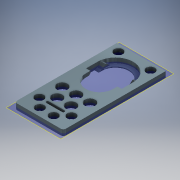
# Autodesk Inventor part: Cup_Dispenser_Slider
Saved by Autodesk Inventor 2016 (Build 200138000, 138)
## iProperties
Created: 2015-07-09
Part Number: Cup_Dispenser_Slider
Material: Generic
Document SubType Name: Modeling
Designer: marku
Density: 1 g/cm^3
Appearance: Lead
Author: marku
Autodesk Inventor part; units mm, degrees
ref_plane "YZ Plane" through (0, 0, 0) normal (1, 0, 0) x (0, 1, 0)
ref_plane "XZ Plane" through (0, 0, 0) normal (0, 1, 0) x (-1, 0, 0)
ref_plane "XY Plane" through (0, 0, 0) normal (0, 0, 1) x (1, 0, 0)
sketch "Sketch2" plane through (0, 0, 0) normal (0, 0, 1) x (1, 0, 0)
  line L0 (57, 57.2078) -> (57, 117.2078) projected
  line L1 (57, -62.7922) -> (57, 57.2078) projected
  line L2 (57, -112.7922) -> (57, -62.7922) projected
  arc A0 (50, -119.7922) -> (57, -112.7922) centre (50, -112.7922) ccw projected
  line L3 (0, -119.7922) -> (50, -119.7922) projected
  line L4 (-50, -119.7922) -> (0, -119.7922) projected
  arc A1 (-57, -112.7922) -> (-50, -119.7922) centre (-50, -112.7922) ccw projected
  line L5 (-57, -62.7922) -> (-57, -112.7922) projected
  line L6 (-57, 57.2078) -> (-57, -62.7922) projected
  line L7 (-57, 117.2078) -> (-57, 57.2078) projected
  line L8 (-57, 117.2078) -> (57, 117.2078) projected
  line L9 (54, 114.2078) -> (54, 57.2078)
  line L10 (54, 57.2078) -> (54, -62.7922)
  line L11 (54, -62.7922) -> (54, -112.7922)
  arc A2 (50, -116.7922) -> (54, -112.7922) centre (50, -112.7922) ccw
  line L12 (50, -116.7922) -> (0, -116.7922)
  line L13 (0, -116.7922) -> (-50, -116.7922)
  arc A3 (-54, -112.7922) -> (-50, -116.7922) centre (-50, -112.7922) ccw
  line L14 (-54, -112.7922) -> (-54, -62.7922)
  line L15 (-54, -62.7922) -> (-54, 57.2078)
  line L16 (-54, 57.2078) -> (-54, 114.2078)
  line L17 (-54, 114.2078) -> (54, 114.2078)
  point P0 (0, 0)
  dimension "d5" = 3
  constraints: 18 end point, 4 point on circle, 2 centre point, 10 other
  measures "d5" distance between parallel lines of L0 L9
ref_plane "Work Plane1" through (-57, -119.7922, 15) normal (0, 0, -1) x (0, 1, 0)
extrude "Extrusion1" add sketch "Sketch2" along normal up to surface (15 mm away)
sketch "Sketch3" plane through (0, 0, 0) normal (0, 0, -1) x (-1, 0, 0)
  circle A0 centre (0, 57.2078) radius 57 construction
  arc A1 (31.25, 57.2078) -> (-31.25, 57.2078) centre (0, 57.2078) ccw
  line L0 (-54, -112.7922) -> (-54, 114.2078) projected
  line L1 (-54, 114.2078) -> (54, 114.2078) projected
  line L2 (54, 114.2078) -> (54, -112.7922) projected
  line L3 (-31.25, 57.2078) -> (-31.25, 47.2078)
  line L4 (-31.25, 47.2078) -> (-54, 47.2078)
  line L5 (31.25, 57.2078) -> (31.25, 47.2078)
  line L6 (31.25, 47.2078) -> (54, 47.2078)
  point P0 (0, 0)
  dimension "d8" = 31.25
  dimension "d9" = 10
  dimension "d10" = 10
  constraints: 8 end point, 4 point on line, 2 perpendicular, 2 point on circle, 1 centre point, 1 coincident, 1 tangent, 1 vertical
  measures "d8" radius of A1
  measures "d9" distance of L3.start L3.end
  measures "d10" distance of L5.start L5.end
extrude "Extrusion2" add sketch "Sketch3" against normal blind 3
ref_plane "Work Plane2" through (0, 0, 6) normal (0, 0, -1) x (-1, 0, 0)
sketch "Sketch4" plane through (0, 0, 6) normal (0, 0, -1) x (-1, 0, 0)
  line L0 (-54, -112.7922) -> (-54, 47.2078) projected
  arc A0 (-54, -112.7922) -> (-50, -116.7922) centre (-50, -112.7922) ccw projected
  line L1 (50, -116.7922) -> (-50, -116.7922) projected
  arc A1 (50, -116.7922) -> (54, -112.7922) centre (50, -112.7922) ccw projected
  line L2 (54, 47.2078) -> (54, -112.7922) projected
  line L3 (0, -163.3413) -> (0, 169.6733) construction
  line L4 (-31.25, 47.2078) -> (-54, 47.2078) construction
  circle A2 centre (0, 20.6666) radius 41 construction
  arc A3 (-31.25, 20.6666) -> (31.25, 20.6666) centre (0, 20.6666) ccw
  line L5 (-31.25, 20.6666) -> (-31.25, 30.6666)
  line L6 (31.25, 20.6666) -> (31.25, 30.6666)
  line L7 (31.25, 30.6666) -> (54, 30.6666)
  line L8 (-31.25, 30.6666) -> (-54, 30.6666)
  point P0 (0, 0)
  dimension "d14" = 82
  dimension "d15" = 10
  dimension "d16" = 31.25
  constraints: 10 end point, 4 point on line, 3 vertical, 2 perpendicular, 2 point on circle, 2 tangent, 1 centre point, 1 coincident, 1 parallel, 3 other
  measures "d15" distance of L5.start L5.end
  measures "d16" radius of A3
extrude "Extrusion3" add sketch "Sketch4" against normal up to surface (9 mm away)
sketch "Sketch5" plane through (0, 0, 3) normal (0, 0, 1) x (1, 0, 0)
  arc A0 (31.25, 57.2078) -> (-31.25, 57.2078) centre (0, 57.2078) ccw projected
  line L0 (31.25, 57.2078) -> (31.25, 47.2078) projected
  line L1 (31.25, 47.2078) -> (54, 47.2078) projected
  line L2 (54, 114.2078) -> (54, 47.2078) projected
  line L3 (-54, 114.2078) -> (54, 114.2078) projected
  line L4 (-54, 47.2078) -> (-54, 114.2078) projected
  line L5 (-54, 47.2078) -> (-31.25, 47.2078) projected
  line L6 (-31.25, 47.2078) -> (-31.25, 57.2078) projected
  arc A1 (41, 57.2078) -> (-41, 57.2078) centre (0, 57.2078) ccw
  line L7 (41, 57.2078) -> (41, 56.9578)
  line L8 (41, 56.9578) -> (44.25, 56.9578)
  line L9 (44.25, 56.9578) -> (44.25, 104.4578)
  line L10 (44.25, 104.4578) -> (-44.25, 104.4578)
  line L11 (-44.25, 104.4578) -> (-44.25, 56.9578)
  line L12 (-44.25, 56.9578) -> (-41, 56.9578)
  line L13 (-41, 56.9578) -> (-41, 57.2078)
  line L14 (-44.25, 56.9578) -> (-54, 56.9578)
  line L15 (44.25, 56.9578) -> (54, 56.9578)
  point P0 (0, 0)
  dimension "d19" = 41
  constraints: 18 end point, 3 point on line, 2 point on circle, 1 centre point, 1 perpendicular, 7 other
  measures "d19" horizontal distance of A0.centre L12.end
extrude "Extrusion4" add sketch "Sketch5" along normal up to surface (12 mm away) contours L15 L9 L10 L11 L14 L4 L3 L2 | L8 L7 A1 L13 L12 L11 L10 L9
sketch "Sketch6" plane through (0, 0, 6) normal (0, 0, -1) x (-1, 0, 0)
  line L0 (-54, -112.7922) -> (-54, 30.6666) projected
  arc A0 (-54, -112.7922) -> (-50, -116.7922) centre (-50, -112.7922) ccw projected
  line L1 (50, -116.7922) -> (-50, -116.7922) projected
  arc A1 (50, -116.7922) -> (54, -112.7922) centre (50, -112.7922) ccw projected
  line L2 (54, 30.6666) -> (54, -112.7922) projected
  line L3 (31.25, 30.6666) -> (54, 30.6666) projected
  line L4 (31.25, 20.6666) -> (31.25, 30.6666) projected
  arc A2 (-31.25, 20.6666) -> (31.25, 20.6666) centre (0, 20.6666) ccw projected
  line L5 (-31.25, 30.6666) -> (-31.25, 20.6666) projected
  line L6 (-54, 30.6666) -> (-31.25, 30.6666) projected
  line L7 (41, 20.6666) -> (41, 20.9166)
  line L8 (41, 20.9166) -> (44.25, 20.9166)
  line L9 (44.25, 20.9166) -> (44.25, -107.0422)
  line L10 (44.25, -107.0422) -> (-44.25, -107.0422)
  line L11 (-44.25, -107.0422) -> (-44.25, 20.9166)
  line L12 (-44.25, 20.9166) -> (-41, 20.9166)
  line L13 (-41, 20.9166) -> (-41, 20.6666)
  arc A3 (-41, 20.6666) -> (41, 20.6666) centre (0, 20.6666) ccw
  line L14 (44.25, 20.9166) -> (54, 20.9166)
  line L15 (-44.25, 20.9166) -> (-54, 20.9166)
  point P0 (0, 0)
  dimension "d22" = 41
  constraints: 18 end point, 3 point on line, 2 point on circle, 1 centre point, 1 perpendicular, 7 other
  measures "d22" distance of A2.centre L7.start
extrude "Extrusion5" add sketch "Sketch6" along normal up to surface (6 mm away) contours L0 L15 L11 L10 L9 L14 L2 A1 L1 A0 | L12 L13 A3 L7 L8 L9 L10 L11
sketch "Sketch7" plane through (0, 0, 0) normal (0, 0, -1) x (-1, 0, 0)
  line L0 (54, 20.9166) -> (41, 20.9166) projected
  line L1 (41, 20.9166) -> (54, 20.9166) projected
  line L2 (54, 56.9578) -> (41, 56.9578) projected
  line L3 (41, 56.9578) -> (54, 56.9578) projected
  line L4 (54, 47.2078) -> (54, 20.9166) projected
  line L5 (54, 56.9578) -> (54, 20.9166)
  line L6 (41, 56.9578) -> (41, 20.9166)
  line L7 (-41, 56.9578) -> (-54, 56.9578) projected
  line L8 (-41, 20.9166) -> (-54, 20.9166) projected
  line L9 (-41, 56.9578) -> (-41, 20.9166)
  line L10 (-54, 20.9166) -> (-54, 47.2078) projected
  line L11 (-54, 56.9578) -> (-54, 20.9166)
  point P0 (0, 0)
  constraints: 8 end point, 2 collinear, 2 vertical
extrude "Extrusion6" add sketch "Sketch7" against normal up to surface (15 mm away)
chamfer "Chamfer1" distance 10 distance2 3 1 edges at (36.125, 47.2078, 3) measured on face at (36.125, 47.7078, 3)
chamfer "Chamfer2" distance 10 distance2 3 1 edges at (-36.125, 47.2078, 3) measured on face at (-36.125, 47.7078, 3)
sketch "Sketch9" plane through (41, 30.6666, 15) normal (-1, 0, 0) x (0, 0, 1)
  line L0 (-15, 16.5412) -> (-12, 26.5412) projected
  line L1 (-12, 26.5412) -> (-12, 67.5412) projected
  line L2 (-12, 26.5412) -> (-4, 36.0753)
  line L3 (-4, 36.0753) -> (-12, 45.6093)
  line L4 (-12, 26.5412) -> (-12, 45.6093)
  line L5 (-4, 36.0753) -> (-12, 36.0753) construction
  point P0 (-15, -30.6666)
  dimension "d41" = 100
  dimension "d42" = 8
  constraints: 8 end point, 1 collinear, 1 midpoint, 1 point on line, 1 other
  measures "d41" angle of L2 L3
  measures "d42" distance from line of L1 L2.end
extrude "Extrusion8" add sketch "Sketch9" along normal up to surface (9.75 mm away)
mirror "Mirror1" about plane through (0, 0, 0) normal (1, 0, 0) of "Extrusion8"
fillet "Fillet1" radius 2 2 edges at (-35.563, 66.7418, 11) (35.563, 66.7418, 11)
chamfer "Chamfer4" distance 3 angle 45 2 edges at (36.125, 30.6666, 6) (-36.125, 30.6666, 6)
sketch "Sketch8" plane through (-57, 117.2078, 15) normal (0, 0, 1) x (1, 0, 0)
  arc A0 (98, -60) -> (16, -60) centre (57, -60) ccw construction
  arc A1 (16, -96.5412) -> (98, -96.5412) centre (57, -96.5412) ccw construction
  line L0 (57, -60) -> (57, -96.5412) construction
  circle A2 centre (57, -180) radius 57 construction
  line L1 (57, -180) -> (142.4239, -180) construction
  line L2 (57, -161.7294) -> (57, -198.2706) construction
  circle A3 centre (57, -180) radius 18.2706 construction
  line L3 (38.7294, -198.2706) -> (75.2706, -198.2706) construction
  line L4 (38.7294, -201.2706) -> (75.2706, -201.2706)
  line L5 (75.2706, -195.2706) -> (38.7294, -195.2706)
  arc A4 (38.7294, -195.2706) -> (38.7294, -201.2706) centre (38.7294, -198.2706) ccw
  arc A5 (75.2706, -201.2706) -> (75.2706, -195.2706) centre (75.2706, -198.2706) ccw
  line L6 (75.2706, -180) -> (75.2706, -198.2706) construction
  point P0 (57, -117.2078)
  dimension "d33" = 6
  constraints: 16 end point, 6 point on circle, 6 tangent, 3 centre point, 2 horizontal, 2 midpoint, 2 vertical, 1 coincident, 1 collinear, 1 parallel, 1 perpendicular, 1 point on line, 1 symmetric about line
  measures "d33" diameter of A5
extrude "Extrusion7" cut sketch "Sketch8" against normal up to surface (15 mm away)
chamfer "Chamfer3" distance 1.5 angle 45 4 edges at (0, -78.0628, 0) (-21.2706, -81.0628, 0) (0, -84.0628, 0) (21.2706, -81.0628, 0)
sketch "Sketch10" plane through (-57, 117.2078, 0) normal (0, 1, 0) x (1, 0, 0)
  line L0 (0, 0) -> (0, -15) projected
  line L1 (0, -7.5) -> (114, -7.5) construction
  line L2 (114, 0) -> (114, -15) projected
  line L3 (57, 0) -> (57, -7.5) construction
  line L4 (57, -7.5) -> (57, -15) construction
  point P0 (15, -7.5)
  point P1 (99, -7.5)
  dimension "d46" = 15
  constraints: 6 end point, 3 midpoint, 2 point on line, 1 symmetric about line
  measures "d46" distance from line of L0 point (15, -7.5)
hole "Hole1" at (-42, 117.2078, 7.5) at (42, 117.2078, 7.5) direction (0, -1, 0) diameter 3 depth 8 tip angle 118
thicken "Thicken1" operation add thickness 0.8 both sides no extend neighbours yes toward (0, 0, -1) faces at (-51.6667, 11.694, 15) (-57, 40.5411, 5) (57, -36.1255, 5) (-50.5231, -119.7726, 10) (-16.6667, -119.7922, 5) (50.5231, -119.7726, 5) (51.6667, 8.3607, 0)
sketch "Sketch11" plane through (-56.2, 117.2078, 14.2) normal (0, 0, 1) x (1, 0, 0)
  circle A0 centre (56.2, -150.5412) radius 12
  line L0 (74.4706, -201.2706) -> (37.9294, -201.2706) construction
  arc A1 (37.9294, -195.2706) -> (37.9294, -201.2706) centre (37.9294, -198.2706) ccw construction
  line L1 (37.9294, -195.2706) -> (74.4706, -195.2706) construction
  arc A2 (74.4706, -201.2706) -> (74.4706, -195.2706) centre (74.4706, -198.2706) ccw construction
  line L2 (112.4, -230) -> (112.4, 0) construction
  line L3 (112.4, 0) -> (0, 0) construction
  line L4 (0, 0) -> (0, -230) construction
  arc A3 (0, -230) -> (6.2, -236.2) centre (6.2, -230) ccw construction
  line L5 (6.2, -236.2) -> (106.2, -236.2) construction
  arc A4 (106.2, -236.2) -> (112.4, -230) centre (106.2, -230) ccw construction
  line L6 (15.2, -86.5412) -> (15.2, -60) construction
  arc A5 (97.2, -60) -> (15.2, -60) centre (56.2, -60) ccw construction
  line L7 (97.2, -60) -> (97.2, -86.5412) construction
  line L8 (97.2, -86.5412) -> (87.45, -86.5412) construction
  line L9 (87.45, -86.5412) -> (87.45, -96.5412) construction
  arc A6 (24.95, -96.5412) -> (87.45, -96.5412) centre (56.2, -96.5412) ccw construction
  line L10 (24.95, -96.5412) -> (24.95, -86.5412) construction
  line L11 (24.95, -86.5412) -> (15.2, -86.5412) construction
  circle A7 centre (88.2, -150.5412) radius 12
  circle A8 centre (24.2, -150.5412) radius 12
  circle A9 centre (72.2, -178.2541) radius 12
  line L12 (56.2, -150.5412) -> (72.2, -178.2541) construction
  line L13 (72.2, -178.2541) -> (88.2, -150.5412) construction
  line L14 (88.2, -150.5412) -> (56.2, -150.5412) construction
  circle A10 centre (40.2, -178.2541) radius 12
  circle A11 centre (93.2, -198.2706) radius 10
  circle A12 centre (19.2, -198.2706) radius 10
  line L15 (56.2, -60) -> (56.2, -293.0623) construction
  circle A13 centre (72.2, -218.2706) radius 10
  line L16 (72.2, -178.2541) -> (72.2, -218.2706) construction
  circle A14 centre (40.2, -218.2706) radius 10
  circle A15 centre (19.2, -16) radius 10
  circle A16 centre (93.2, -16) radius 10
  line L17 (93.2, -16) -> (93.2, -198.2706) construction
  arc A17 (74.4706, -201.2706) -> (74.4706, -195.2706) centre (74.4706, -198.2706) ccw construction
  line L18 (93.2, -198.2706) -> (74.4706, -198.2706) construction
  point P0 (56.2, -117.2078)
  dimension "d56" = 24
  dimension "d59" = 32
  dimension "d66" = 32
  dimension "d71" = 24
  dimension "d74" = 32
  dimension "d79" = 20
  dimension "d80" = 20
  dimension "d81" = 20
  dimension "d82" = 20
  dimension "d83" = 5
  dimension "d84" = 16
  dimension "d85" = 54
  dimension "d86" = 20
  constraints: 14 end point, 11 centre point, 5 horizontal, 3 symmetric about line, 3 vertical, 2 equal length, 1 point on line, 8 other
  measures "d56" diameter of A0
  measures "d59" distance of L12.start L13.end
  measures "d66" distance of L12.start A8.centre
  measures "d71" diameter of A9
  measures "d74" distance of L12.end A10.centre
  measures "d79" diameter of A11
  measures "d80" diameter of A12
  measures "d81" diameter of A13
  measures "d82" diameter of A15
  measures "d83" distance from line of L13.end L17
  measures "d84" distance from line of L3 L17.start
  measures "d85" distance of A6.centre L12.start
  measures "d86" vertical distance of L16.end A2.centre
extrude "Extrusion9" cut sketch "Sketch11" against normal up to surface (13.4 mm away)
equation "\"d5\" = thickness"
equation "\"d8\" = cup_small_radius"
equation "\"d9\" = elongation"
equation "\"d10\" = d9"
equation "\"d11\" = thickness"
equation "\"d14\" = 2 * radius_tolerance + 2 * cup_big_radius"
equation "\"d15\" = elongation"
equation "\"d16\" = cup_small_radius"
equation "\"d17\" = thickness"
equation "\"d19\" = cup_big_radius + radius_tolerance"
equation "\"d20\" = thickness"
equation "\"d22\" = cup_big_radius + radius_tolerance"
equation "\"d23\" = thickness"
equation "\"d25\" = thickness"
equation "\"d27\" = elongation"
equation "\"d28\" = thickness"
equation "\"d30\" = elongation"
equation "\"d31\" = thickness"
equation "\"d42\" = 4 * cup_gap"
equation "\"d43\" = thickness"
equation "\"d89\" = thickness"
equation "\"d90\" = thickness"
equation "\"d33\" = 2 * thickness"
equation "\"d34\" = thickness"
equation "\"d36\" = 0.5 * thickness"
equation "\"d37\" = thickness"
equation "\"d46\" = 5 * thickness"
equation "\"d87\" = thickness"
equation "\"thickness\" = 3"
equation "\"cup_to_cup_distance\" = 4"
equation "\"cup_lid_end_height\" = 2"
equation "\"cup_gap\" = 2"
equation "\"cup_lid_height\" = 5"
equation "\"cup_small_radius\" = 31.25"
equation "\"cup_big_radius\" = 39"
equation "\"elongation\" = 10"
equation "\"d13\" = -0.5 * cup_gap - cup_lid_height"
equation "\"radius_tolerance\" = 2"
equation "\"bearing_tolerance\" = 1"
body "Solid1"
